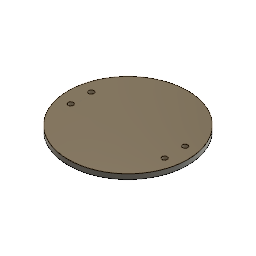
ボード v1 (Autodesk Fusion 360 design; units mm, degrees)
Autodesk Fusion 360 part; units mm, degrees
sketch "スケッチ1" plane through (0, 0, 0) normal (1, 0, 0) x (0, 0, -1)
sketch "スケッチ2" plane through (0, 0, 0) normal (0, 1, 0) x (1, 0, 0)
  circle A0 centre (0, 0) radius 35
  dimension "d1" = 70
  measures "d1" diameter of A0
extrude "押し出し1" add sketch "スケッチ2" along normal blind 3
sketch "スケッチ3" plane through (0, 3, 0) normal (0, 1, 0) x (-1, 0, 0)
  circle A0 centre (0, 0) radius 35
  line L0 (35, 0) -> (-35, 0)
  circle A1 centre (-27.5, -6) radius 1.5
  circle A2 centre (-27.5, 6) radius 1.5
  circle A3 centre (27.5, -6) radius 1.5
  circle A4 centre (27.5, 6) radius 1.5
  point P0 (0, -0.0001)
  dimension "d4" = 3
  dimension "d5" = 27.5
  dimension "d6" = 6
  dimension "d7" = 3
  dimension "d8" = 6
  dimension "d9" = 27.5
  dimension "d10" = 3
  dimension "d11" = 3
  dimension "d12" = 27.5
  dimension "d13" = 27.5
  dimension "d14" = 6
  dimension "d15" = 6
  measures "d4" diameter of A1
  measures "d5" distance of A0.centre
  measures "d7" diameter of A2
  measures "d9" distance of A0.centre
  measures "d10" diameter of A3
  measures "d11" diameter of A4
  measures "d12" distance of A0.centre
  measures "d13" distance of A0.centre
extrude "押し出し2" cut sketch "スケッチ3" along normal mid plane 6 contours A1 | A2 | A3 | A4
sketch "スケッチ4" plane through (0, 3, 0) normal (0, 1, 0) x (-1, 0, 0)
  circle A0 centre (27.5, 6) radius 1.5
  circle A1 centre (-27.5, -6) radius 1.5
  circle A2 centre (27.5, -6) radius 1.5
  circle A3 centre (-27.5, 6) radius 1.5
  circle A4 centre (0, 0) radius 35
equation "d5 = ( 55 / 2 ) * 1 mm"
